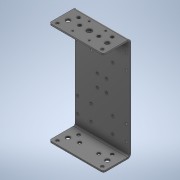
# Autodesk Inventor part: De  truc Y
Saved by Autodesk Inventor 2020 (Build 240168000, 168)
## iProperties
Created: 2021-05-26
Part Number: De  truc Y
Material: Generic
Document SubType Name: Sheet Metal
Designer: admin
Density: 1 g/cm^3
Sheet Metal Rule: Default_mm
Appearance: Smooth - Black
Author: admin
Autodesk Inventor part; units mm, degrees
ref_plane "YZ Plane" through (0, 0, 0) normal (1, 0, 0) x (0, 1, 0)
ref_plane "XZ Plane" through (0, 0, 0) normal (0, 1, 0) x (-1, 0, 0)
ref_plane "XY Plane" through (0, 0, 0) normal (0, 0, 1) x (1, 0, 0)
sketch "Sketch1" plane through (0, 0, 0) normal (0, 0, 1) x (1, 0, 0)
  line L0 (-52.5, -100) -> (52.5, -100)
  line L1 (52.5, -100) -> (52.5, 100)
  line L2 (52.5, 100) -> (-52.5, 100)
  line L3 (-52.5, 100) -> (-52.5, -100)
  line L4 (-52.5, -100) -> (52.5, 100) construction
  line L5 (52.5, -100) -> (-52.5, 100) construction
  point P0 (0, 0)
  dimension "d0" = 105
  dimension "d1" = 200
  measures "d0" distance of L2.end L1.end
  measures "d1" distance of L1.end L0.end
extrude "Plate1" add sketch "Sketch1" along normal blind 3
sketch "Sketch2" plane through (-52.5, 97, 0) normal (0, 1, 0) x (-1, 0, 0)
  line L0 (-105, 0) -> (0, 0)
  line L1 (0, 0) -> (0, 53)
  line L2 (0, 53) -> (-105, 53)
  line L3 (-105, 53) -> (-105, 0)
  constraints: 6 end point, 1 horizontal, 1 perpendicular, 1 vertical
edge flange "Flange1" height 53 angle 90 thickness 3 bend radius 3 thickness toward (0, 1, 0) relief tear relief width 3 relief depth 1.5 corner gap 3 corner form 0 edges at (0, 100, 3) (0, -100, 3) wall of the first edge with corners at (52.5, 97, 0) (-52.5, 97, 0) (-52.5, 97, 53) (52.5, 97, 53)
bend "Bend1"
corner "Corner1"
sketch "Sketch3" plane through (-52.5, 100, 53) normal (0, 1, 0) x (1, 0, 0)
  circle A0 centre (14.5, 22) radius 4.15
  circle A1 centre (90.5, 22) radius 4.15
  line L0 (105, 0) -> (0, 0) projected
  point P0 (52.5, 53)
  dimension "d13" = 8.3
  dimension "d14" = 8.3
  dimension "d15" = 76
  dimension "d16" = 38
  dimension "d17" = 22
  dimension "d18" = 22
  constraints: 2 centre point
  measures "d13" diameter of A0
  measures "d14" diameter of A1
  measures "d15" distance of A1.centre A0.centre
  measures "d16" horizontal distance of A0.centre point (52.5, 53)
  measures "d17" distance from line of L0 A0.centre
  measures "d18" distance from line of L0 A1.centre
extrude "Cut1" cut sketch "Sketch3" against normal through all
sketch "Sketch4" plane through (-52.5, -100, 53) normal (0, -1, 0) x (1, 0, 0)
  circle A0 centre (71, -25) radius 3.25
  circle A1 centre (34, -25) radius 3.25
  line L0 (0, 0) -> (105, 0) projected
  point P0 (52.5, -53)
  dimension "d21" = 37
  dimension "d22" = 18.5
  dimension "d23" = 6.5
  dimension "d24" = 6.5
  dimension "d25" = 25
  dimension "d26" = 25
  constraints: 2 centre point
  measures "d21" distance of A1.centre A0.centre
  measures "d22" horizontal distance of point (52.5, -53) A0.centre
  measures "d23" diameter of A0
  measures "d24" diameter of A1
  measures "d25" distance from line of L0 A0.centre
  measures "d26" distance from line of L0 A1.centre
extrude "Cut2" cut sketch "Sketch4" against normal blind 3
fillet "Fillet1" radius 4 4 edges at (-52.5, -98.5, 53) (52.5, -98.5, 53) (52.5, 98.5, 53) (-52.5, 98.5, 53)
sketch "Sketch5" plane through (-52.5, 100, 6) normal (0, 1, 0) x (1, 0, 0)
  line L0 (36.5, -38) -> (68.5, -38)
  line L1 (68.5, -38) -> (68.5, -6)
  line L2 (68.5, -6) -> (36.5, -6)
  line L3 (36.5, -6) -> (36.5, -38)
  line L4 (36.5, -38) -> (68.5, -6) construction
  line L5 (68.5, -38) -> (36.5, -6) construction
  line L6 (101, -47) -> (4, -47) projected
  circle A0 centre (36.5, -38) radius 1.75
  circle A1 centre (68.5, -38) radius 1.75
  circle A2 centre (68.5, -6) radius 1.75
  circle A3 centre (36.5, -6) radius 1.75
  circle A4 centre (52.5, -22) radius 5
  circle A5 centre (34, -22) radius 3.25
  circle A6 centre (71, -22) radius 3.25
  point P0 (52.5, 6)
  dimension "d30" = 32
  dimension "d31" = 32
  dimension "d32" = 0
  dimension "d33" = 25
  dimension "d34" = 3.5
  dimension "d35" = 3.5
  dimension "d36" = 3.5
  dimension "d37" = 3.5
  dimension "d38" = 10
  dimension "d41" = 6.5
  dimension "d42" = 6.5
  dimension "d43" = 25
  dimension "d44" = 25
  dimension "d45" = 37
  dimension "d46" = 18.5
  constraints: 12 end point, 7 centre point, 5 coincident, 2 midpoint, 2 parallel, 1 horizontal, 1 perpendicular
  measures "d30" distance between parallel lines of L0 L2
  measures "d31" distance between parallel lines of L1 L3
  measures "d32" horizontal distance of point (52.5, -22) point (52.5, 6)
  measures "d33" distance from line of L6 point (52.5, -22)
  measures "d34" diameter of A0
  measures "d35" diameter of A1
  measures "d36" diameter of A2
  measures "d37" diameter of A3
  measures "d38" diameter of A4
  measures "d41" diameter of A5
  measures "d42" diameter of A6
  measures "d43" distance from line of L6 A6.centre
  measures "d44" distance from line of L6 A5.centre
  measures "d45" distance of A6.centre A5.centre
  measures "d46" horizontal distance of point (52.5, 6) A5.centre
extrude "Cut3" cut sketch "Sketch5" against normal blind 3 contours L3 A0 L0 | L0 A0 L3 | A1 L1 L0 | L0 L1 A1 | A5 L3 | L3 A5 | A6 L1 | L1 A6 | A3 L2 L3 | L3 L2 A3 | A2 L2 L1 | L1 L2 A2 | A4
sketch "Sketch6" plane through (0, 0, 0) normal (0, 0, -1) x (-1, 0, 0)
  line L0 (47, 75.25) -> (21, 75.25)
  circle A0 centre (47, 75.25) radius 2.25
  circle A1 centre (21, 75.25) radius 2.25
  line L1 (47, 44.75) -> (47, 75.25)
  line L2 (47, 44.75) -> (21, 75.25) construction
  line L3 (21, 75.25) -> (21, 44.75)
  line L4 (21, 44.75) -> (47, 44.75)
  line L5 (47, 75.25) -> (21, 44.75) construction
  circle A2 centre (47, 44.75) radius 2.25
  circle A3 centre (21, 44.75) radius 2.25
  line L6 (73.5, 0) -> (-73.5, 0) projected
  line L7 (0, -140) -> (0, 140) projected
  point P0 (0, 0)
  point P1 (34, 60)
  dimension "d47" = 30.5
  dimension "d48" = 26
  dimension "d49" = 4.5
  dimension "d50" = 4.5
  dimension "d51" = 4.5
  dimension "d52" = 4.5
  dimension "d53" = 60
  dimension "d54" = 34
  constraints: 12 end point, 4 centre point, 4 coincident, 3 parallel, 2 midpoint, 1 perpendicular
  measures "d47" distance of L3.end L0.end
  measures "d48" distance of L0.end L0.start
  measures "d49" diameter of A1
  measures "d50" diameter of A0
  measures "d51" diameter of A2
  measures "d52" diameter of A3
  measures "d53" vertical distance of point (0, 0) point (34, 60)
  measures "d54" horizontal distance of point (0, 0) point (34, 60)
extrude "Cut4" cut sketch "Sketch6" against normal blind 3 contours A1 L3 L0 | L0 L3 A1 | A0 L1 L0 | L0 L1 A0 | A3 L4 L3 | L3 L4 A3 | A2 L4 L1 | L1 L4 A2
pattern_linear "Rectangular Pattern1" count 2 spacing 68 along (1, 0, 0) count 2 spacing 120 along (0, -1, 0) of "Cut4"
sketch "Sketch7" plane through (0, 0, 0) normal (0, 0, -1) x (-1, 0, 0)
  line L0 (9, -12) -> (9, 12)
  line L1 (9, 12) -> (-9, 12)
  line L2 (-9, 12) -> (-9, -12)
  line L3 (-9, -12) -> (9, -12)
  line L4 (9, -12) -> (-9, 12) construction
  line L5 (9, 12) -> (-9, -12) construction
  circle A0 centre (-9, -12) radius 2.25
  circle A1 centre (-9, 12) radius 2.25
  circle A2 centre (9, 12) radius 2.25
  circle A3 centre (9, -12) radius 2.25
  point P0 (0, 0)
  point P1 (0, 0)
  dimension "d63" = 24
  dimension "d64" = 18
  dimension "d65" = 4.5
  dimension "d66" = 4.5
  dimension "d67" = 4.5
  dimension "d68" = 4.5
  constraints: 12 end point, 4 centre point, 4 coincident, 2 midpoint, 2 parallel, 1 perpendicular
  measures "d63" distance of L2.end L1.end
  measures "d64" distance of L1.end L1.start
  measures "d65" diameter of A0
  measures "d66" diameter of A1
  measures "d67" diameter of A2
  measures "d68" diameter of A3
extrude "Cut5" cut sketch "Sketch7" against normal blind 3 contours L3 A3 L0 | L0 A3 L3 | A2 L1 L0 | L0 L1 A2 | A0 L2 L3 | L3 L2 A0 | A1 L2 L1 | L1 L2 A1
sketch "Sketch8" plane through (-52.5, 100, 6) normal (0, 1, 0) x (1, 0, 0)
  circle A0 centre (14.5, -25) radius 4.15 projected
  line L0 (14.5, -25) -> (19.9723, -9.9649)
  line L1 (14.5, -25) -> (30.5, -25) construction
  line L2 (14.5, -25) -> (9.0277, -40.0351)
  line L3 (14.5, -25) -> (30.5, -25) construction
  circle A1 centre (9.0277, -40.0351) radius 3
  circle A2 centre (19.9723, -9.9649) radius 3
  circle A3 centre (90.5, -25) radius 4.15 projected
  line L4 (90.5, -25) -> (85.0277, -9.9649)
  line L5 (90.5, -25) -> (106.5, -25) construction
  line L6 (90.5, -25) -> (95.9723, -40.0351)
  line L7 (90.5, -25) -> (106.5, -25) construction
  line L8 (52.5, 16.6) -> (52.5, -57.6) projected
  circle A4 centre (95.9723, -40.0351) radius 3
  circle A5 centre (85.0277, -9.9649) radius 3
  point P0 (52.5, 6)
  dimension "d71" = 16
  dimension "d72" = 70
  dimension "d73" = 16
  dimension "d74" = 110
  dimension "d75" = 6
  dimension "d76" = 6
  dimension "d77" = 16
  dimension "d78" = 110
  dimension "d79" = 16
  dimension "d80" = 70
  dimension "d81" = 6
  dimension "d82" = 6
  constraints: 16 end point, 4 centre point, 4 coincident, 4 equal length, 4 horizontal
  measures "d71" distance of L0.start L0.end
  measures "d72" angle of L1 L0
  measures "d73" distance of L0.start L2.end
  measures "d74" angle of L2 L3
  measures "d75" diameter of A1
  measures "d76" diameter of A2
  measures "d77" distance of L4.start L4.end
  measures "d78" angle of L5 L4
  measures "d79" distance of L4.start L6.end
  measures "d80" angle of L6 L7
  measures "d81" diameter of A4
  measures "d82" diameter of A5
extrude "Cut6" cut sketch "Sketch8" against normal through all contours A1 | A2 | A4 | A5
equation "\"d19\" = Thickness"
equation "\"d27\" = Thickness"
equation "\"d39\" = Thickness"
equation "\"d55\" = Thickness"
equation "\"d69\" = Thickness"
equation "\"d83\" = Thickness"
equation "\"d2\" = Thickness"
equation "\"d3\" = BendReliefWidth"
equation "\"d4\" = BendReliefDepth"
equation "\"d5\" = MinimumRemnant"
equation "\"d6\" = TransitionRadius"
equation "\"d9\" = BendRadius"
equation "\"d10\" = CornerReliefSize"
equation "\"d11\" = GapSize"
equation "\"d12\" = JacobiRadiusSize"
equation "\"BendRadius\" = Thickness"
equation "\"BendReliefWidth\" = Thickness"
equation "\"BendReliefDepth\" = 0.5 * Thickness"
equation "\"CornerReliefSize\" = 4 * Thickness"
equation "\"MinimumRemnant\" = 2 * Thickness"
equation "\"TransitionRadius\" = BendRadius"
equation "\"JacobiRadiusSize\" = BendRadius"
equation "\"GapSize\" = Thickness"
equation "\"Thickness\" = 3"
body "Solid1"
